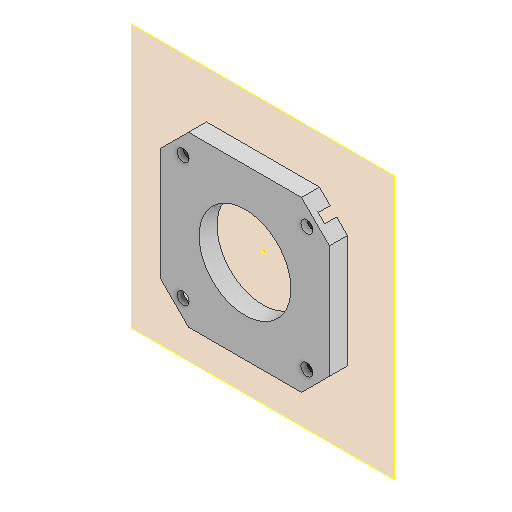
# Autodesk Inventor part: 55_spiralxy_motorplate_nema_mgn9
Saved by Autodesk Inventor 2022 (Build 260153000, 153)
## iProperties
Created: 2023-09-18
Part Number: 55_spiralxy_motorplate_nema_mgn9
Material: Generisch
Document SubType Name: Modeling
Designer: diederichbenedict
Density: 1 g/cm^3
Appearance: Vorgabe
Author: diederichbenedict
Autodesk Inventor part; units mm, degrees
ref_plane "YZ Plane" through (0, 0, 0) normal (1, 0, 0) x (0, 1, 0)
ref_plane "XZ Plane" through (0, 0, 0) normal (0, 1, 0) x (-1, 0, 0)
ref_plane "XY Plane" through (0, 0, 0) normal (0, 0, 1) x (1, 0, 0)
ref_plane "Arbeitsebene1" through (0, 0, 0) normal (0, 0, 1) x (1, 0, 0)
sketch "Skizze1" plane through (0, 0, 0) normal (0, 0, 1) x (1, 0, 0)
  circle A0 centre (0, 0) radius 7.5 projected
  circle A1 centre (15.5, -15.5) radius 1.5 projected
  circle A2 centre (-15.5, -15.5) radius 1.5 projected
  circle A3 centre (-15.5, 15.5) radius 1.5 projected
  circle A4 centre (15.5, 15.5) radius 1.5 projected
  line L0 (21.15, 14.15) -> (21.15, -14.15) projected
  line L1 (14.15, 21.15) -> (21.15, 14.15) projected
  line L2 (-14.15, 21.15) -> (14.15, 21.15) projected
  line L3 (-21.15, 14.15) -> (-14.15, 21.15) projected
  line L4 (-21.15, -14.15) -> (-21.15, 14.15) projected
  line L5 (-14.15, -21.15) -> (-21.15, -14.15) projected
  line L6 (14.15, -21.15) -> (-14.15, -21.15) projected
  line L7 (21.15, -14.15) -> (14.15, -21.15) projected
  line L8 (-21, 16) -> (-16, 21) projected
  line L9 (-21, 16) -> (-21, -16) projected
  line L10 (-16, -21) -> (16, -21) projected
  line L11 (21, -16) -> (16, -21) projected
  line L12 (21, -16) -> (21, 16) projected
  line L13 (16, 21) -> (21, 16) projected
  line L14 (16, 21) -> (-16, 21) projected
  circle A5 centre (0, 15.5563) radius 2.6 projected
  circle A6 centre (0, -15.5563) radius 2.6 projected
  circle A7 centre (-15.5563, 0) radius 2.6 projected
  circle A8 centre (15.5563, 0) radius 2.6 projected
  line L15 (-16, -21) -> (-21, -16) projected
  circle A9 centre (0, 0) radius 11.5
  point P0 (0, 0)
  dimension "d17" = 23
  constraints: 1 centre point, 1 coincident
  measures "d17" diameter of A9
extrude "Extrusion1" add sketch "Skizze1" along normal blind 4.5 contours L0 L7 L12 L1 | L12 L7 L10 L5 L9 L3 L14 L1 | L14 L3 L2 L1 | L7 L6 L5 L10 | L9 L5 L4 L3 | A5 | A6 | A7 | A8
sketch "Skizze2" plane through (0, 0, 0) normal (0, 0, -1) x (-1, 0, 0)
  circle A0 centre (15.5, -15.5) radius 1.5 projected
  circle A1 centre (15.5, 15.5) radius 1.5 projected
  circle A2 centre (-15.5, 15.5) radius 1.5 projected
  circle A3 centre (-15.5, -15.5) radius 1.5 projected
  point P0 (0, 0)
hole "Bohrung1" at (15.5, -15.5, 0) at (-15.5, -15.5, 0) at (-15.5, 15.5, 0) at (15.5, 15.5, 0) direction (0, 0, 1) diameter 2.8 end through all counterbore diameter 6.5 counterbore depth 3
sketch "Skizze3" plane through (0, 0, 0) normal (0, 0, -1) x (-1, 0, 0)
  point P0 (0, 0)
sketch "Skizze4" plane through (0, 0, 0) normal (0, 0, -1) x (-1, 0, 0)
  arc A0 (16.8384, 18.4616) -> (18.4616, 16.8384) centre (15.5, 15.5) ccw projected
  line L0 (14.15, 21.15) -> (16.8384, 18.4616) projected
  line L1 (-14.15, 21.15) -> (14.15, 21.15) projected
  line L2 (-16.8384, 18.4616) -> (-14.15, 21.15) projected
  arc A1 (-18.4616, 16.8384) -> (-16.8384, 18.4616) centre (-15.5, 15.5) ccw projected
  line L3 (-21.15, 14.15) -> (-18.4616, 16.8384) projected
  line L4 (-21.15, -14.15) -> (-21.15, 14.15) projected
  line L5 (-18.4616, -16.8384) -> (-21.15, -14.15) projected
  arc A2 (-16.8384, -18.4616) -> (-18.4616, -16.8384) centre (-15.5, -15.5) ccw projected
  line L6 (-14.15, -21.15) -> (-16.8384, -18.4616) projected
  line L7 (14.15, -21.15) -> (-14.15, -21.15) projected
  line L8 (16.8384, -18.4616) -> (14.15, -21.15) projected
  arc A3 (18.4616, -16.8384) -> (16.8384, -18.4616) centre (15.5, -15.5) ccw projected
  line L9 (21.15, -14.15) -> (18.4616, -16.8384) projected
  line L10 (21.15, 14.15) -> (21.15, -14.15) projected
  line L11 (18.4616, 16.8384) -> (21.15, 14.15) projected
  line L12 (0, -15.5563) -> (15.5563, 0)
  line L13 (15.5563, 0) -> (0, 15.5563)
  line L14 (0, 15.5563) -> (-15.5563, 0)
  line L15 (-15.5563, 0) -> (0, -15.5563)
  line L16 (0, -15.5563) -> (0, 15.5563) construction
  line L17 (15.5563, 0) -> (-15.5563, 0) construction
  circle A4 centre (15.5563, 0) radius 2.5
  circle A5 centre (0, -15.5563) radius 2.5
  circle A6 centre (-15.5563, 0) radius 2.5
  circle A7 centre (0, 15.5563) radius 2.5
  point P0 (0, 0)
  dimension "d9" = 22
  dimension "d10" = 22
  dimension "d11" = 5
  dimension "d12" = 5
  dimension "d13" = 5
  dimension "d14" = 5
  constraints: 12 end point, 4 centre point, 4 coincident, 2 parallel, 1 perpendicular
  measures "d9" distance of L12.start L12.end
  measures "d10" distance of L13.end L12.end
  measures "d11" diameter of A4
  measures "d12" diameter of A5
  measures "d13" diameter of A6
  measures "d14" diameter of A7
extrude "Extrusion2" add sketch "Skizze4" along normal blind 1 contours L15 A5 L12 | L12 A5 L15 | A4 L13 L12 | L12 L13 A4 | A6 L14 L15 | L15 L14 A6 | A7 L14 L13 | L13 L14 A7
